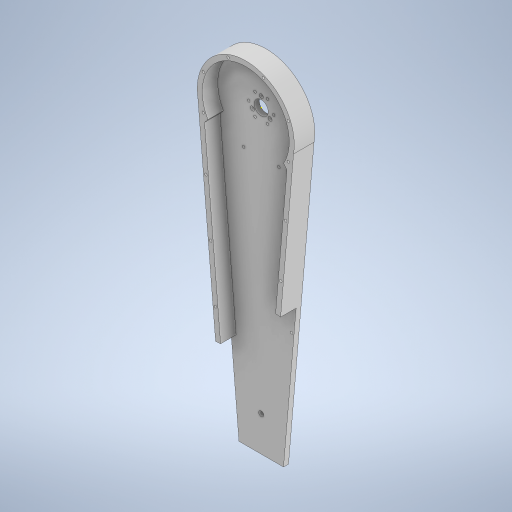
# Autodesk Inventor part: legparts_05(second)
Saved by Autodesk Inventor 2024.3 (Build 283343000, 343)
## iProperties
Created: 2024-10-20
Part Number: legparts_05(second)
Material: 一般
Document SubType Name: Modeling
Designer: 佐藤智貴
Density: 1 g/cm^3
Appearance: 既定
Author: 佐藤智貴
Autodesk Inventor part; units mm, degrees
ref_plane "YZ Plane" through (0, 0, 0) normal (1, 0, 0) x (0, 1, 0)
ref_plane "XZ Plane" through (0, 0, 0) normal (0, 1, 0) x (-1, 0, 0)
ref_plane "XY Plane" through (0, 0, 0) normal (0, 0, 1) x (1, 0, 0)
sketch "スケッチ1" plane through (0, 0, 0) normal (0, 0, 1) x (1, 0, 0)
  circle A0 centre (0, 0) radius 48.5
  circle A1 centre (0, 0) radius 7
  dimension "d0" = 97
  dimension "d1" = 14
  constraints: 2 centre point, 1 coincident
  measures "d0" diameter of A0
  measures "d1" diameter of A1
extrude "押し出し1" add sketch "スケッチ1" along normal blind 20.5
sketch "スケッチ2" plane through (0, 0, 20.5) normal (0, 0, 1) x (1, 0, 0)
  circle A0 centre (0, 0) radius 46
  line L0 (0, 0) -> (0, 59.211)
  line L1 (0, 0) -> (-21.8609, 52.777)
  line L2 (0, 0) -> (27.8226, 47.8581)
  point P0 (-17.6034, 42.4985)
  point P1 (-42.4985, 17.6034)
  point P2 (-42.4985, -17.6034)
  point P3 (-17.6034, -42.4985)
  point P4 (17.6034, -42.4985)
  point P5 (42.4985, -17.6034)
  point P6 (42.4985, 17.6034)
  point P7 (17.6034, 42.4985)
  dimension "d4" = 92
  dimension "d5" = 22.5
  dimension "d8" = 360
  constraints: 6 end point, 1 coincident, 1 point on line, 1 vertical, 12 other
  measures "d5" angle of L1 L0
hole "穴1" at (-17.6034, 42.4985, 20.5) at (-42.4985, 17.6034, 20.5) at (-42.4985, -17.6034, 20.5) at (-17.6034, -42.4985, 20.5) at (17.6034, -42.4985, 20.5) at (42.4985, -17.6034, 20.5) at (42.4985, 17.6034, 20.5) at (17.6034, 42.4985, 20.5) direction (0, 0, -1) diameter 2.459 end through all
sketch "スケッチ3" plane through (0, 0, 20.5) normal (0, 0, 1) x (1, 0, 0)
  circle A0 centre (0, 0) radius 43.5
  dimension "d17" = 87
  constraints: 1 centre point, 1 coincident
  measures "d17" diameter of A0
extrude "押し出し2" cut sketch "スケッチ3" against normal blind 15.5
sketch "スケッチ4" plane through (0, 0, 0) normal (0, 0, -1) x (-1, 0, 0)
  line L0 (0, 0) -> (0, -80.557)
  circle A0 centre (0, 0) radius 48.5 projected
  line L1 (-48.5, 0) -> (-48.5, -300)
  line L2 (48.5, 0) -> (48.5, -300)
  line L3 (-48.5, -300) -> (48.5, -300)
  line L4 (-48.5, 0) -> (-22.2534, -300)
  line L5 (48.5, 0) -> (22.2534, -300)
  point P0 (48.5, 0)
  point P1 (47.7632, -8.4219)
  point P2 (-47.7632, -8.4219)
  dimension "d21" = 48.5
  dimension "d23" = 97
  dimension "d24" = 300
  dimension "d25" = 300
  dimension "d56" = 0
  dimension "d89" = 85
  dimension "d90" = 85
  constraints: 12 end point, 2 point on line, 1 perpendicular, 1 vertical, 2 other
  measures "d21" distance from line of L1 L0.start
  measures "d23" distance between parallel lines of L2 L1
  measures "d24" distance of L2.start L2.end
  measures "d25" distance of L1.start L1.end
  measures "d56" angle of L2 L0
  measures "d89" angle of L3 L5
  measures "d90" angle of L3 L4
extrude "押し出し3" add sketch "スケッチ4" against normal blind 5 contours L5 L3 L4 A0
sketch "スケッチ5" plane through (0, 0, 5) normal (0, 0, 1) x (1, 0, 0)
  line L0 (-48.5, 0) -> (48.5, 0)
  line L1 (-22.2534, -300) -> (22.2534, -300) projected
  circle A0 centre (0, 0) radius 48.5 projected
  circle A1 centre (0, 0) radius 43.5 projected
  line L2 (-47.7632, -8.4219) -> (-22.2534, -300) projected
  line L3 (-48.5, 0) -> (-22.2534, -300)
  line L4 (47.7632, -8.4219) -> (22.2534, -300) projected
  line L5 (-22.2534, -300) -> (22.2534, -300)
  line L6 (22.2534, -300) -> (48.5, 0)
  line L7 (-42.8152, -7.6095) -> (-17.6717, -295)
  line L8 (-17.6717, -295) -> (17.6717, -295)
  line L9 (17.6717, -295) -> (42.7822, -7.9862)
  circle A2 centre (0, 0) radius 48.5
  point P0 (0, -300)
  point P1 (0, -295)
  point P2 (0, -300)
  point P3 (-30.2435, -151.3047)
  point P4 (-41.2491, -25.5101)
  point P5 (41.2491, -25.5101)
  dimension "d33" = 5
  dimension "d91" = 5
  constraints: 14 end point, 3 collinear, 2 midpoint, 1 centre point, 1 coincident, 1 concentric, 2 other
  measures "d33" radial gap between concentric circles of A0 A1
  measures "d91" distance from line of L2 point (-30.243, -151.305)
extrude "押し出し4" add sketch "スケッチ5" along normal blind 15.5 contours L4 L1 L2 A0 L7 L8 L9
sketch "スケッチ6" plane through (0, 0, 20.5) normal (0, 0, 1) x (1, 0, 0)
  line L0 (-22.2534, -300) -> (22.2534, -300) projected
  arc A0 (47.7632, -8.4219) -> (-47.7632, -8.4219) centre (0, 0) ccw projected
  line L1 (-17.6717, -295) -> (-41.2491, -25.5101) projected
  line L2 (41.2491, -25.5101) -> (17.6717, -295) projected
  point P0 (39.8662, -70)
  point P1 (-39.8662, -70)
  point P2 (35.0727, -124.7907)
  point P3 (-35.0727, -124.7907)
  point P4 (30.2791, -179.5814)
  point P5 (-30.2791, -179.5814)
  point P6 (0, -300)
  point P7 (0, 48.5)
  point P8 (48.5, 0)
  dimension "d36" = 348.5
  dimension "d38" = 55
  dimension "d39" = 55
  dimension "d44" = 55
  dimension "d45" = 55
  dimension "d87" = 70
  dimension "d88" = 70
  dimension "d92" = 2.5
  dimension "d93" = 2.5
  dimension "d94" = 2.5
  dimension "d95" = 2.5
  dimension "d96" = 2.5
  dimension "d97" = 2.5
  constraints: 1 midpoint, 1 point on circle
  measures "d36" distance of point (0, -300) point (0, 48.5)
  measures "d38" distance of point (-30.279, -179.581) point (-35.073, -124.791)
  measures "d39" distance of point (-35.073, -124.791) point (-39.866, -70)
  measures "d44" distance of point (30.279, -179.581) point (35.073, -124.791)
  measures "d45" distance of point (39.866, -70) point (35.073, -124.791)
  measures "d87" vertical distance of point (-39.866, -70) point (0, 0)
  measures "d88" vertical distance of point (0, 0) point (39.866, -70)
  measures "d92" distance from line of L1 point (-39.866, -70)
  measures "d93" distance from line of L1 point (-35.073, -124.791)
  measures "d94" distance from line of L1 point (-30.279, -179.581)
  measures "d95" distance from line of L2 point (30.279, -179.581)
  measures "d96" distance from line of L2 point (35.073, -124.791)
  measures "d97" distance from line of L2 point (39.866, -70)
hole "穴2" at (39.8662, -70, 20.5) at (-39.8662, -70, 20.5) at (35.0727, -124.7907, 20.5) at (-35.0727, -124.7907, 20.5) at (30.2791, -179.5814, 20.5) at (-30.2791, -179.5814, 20.5) direction (0, 0, -1) diameter 2.459 end through all
sketch "スケッチ7" plane through (0, 0, 5) normal (0, 0, 1) x (1, 0, 0)
  line L0 (43.5, 0) -> (43.5, -295) projected
  line L1 (43.5, -295) -> (-43.5, -295) projected
  point P0 (0, 0)
  point P1 (0, -265)
  point P2 (48.5, 0)
  dimension "d57" = 43.5
  dimension "d58" = 30
  measures "d57" distance from line of point (0, -265) L0
  measures "d58" distance from line of L1 point (0, -265)
hole "穴3" at (0, -265, 5) direction (0, 0, -1) diameter 5 end through all
sketch "スケッチ12" plane through (0, 0, 20.5) normal (0, 0, 1) x (1, 0, 0)
  circle A0 centre (0, 0) radius 43.5
  circle A1 centre (0, 0) radius 48.5
  line L0 (-41.2491, -25.5101) -> (-17.6717, -295) projected
  line L1 (-41.2491, -25.5101) -> (-37.8431, -21.4511)
  line L2 (17.6717, -295) -> (41.2491, -25.5101) projected
  line L3 (41.2491, -25.5101) -> (37.8431, -21.4511)
  line L4 (-25.9514, -200.3636) -> (-17.1404, -301.073)
  line L5 (-22.2534, -300) -> (-47.7632, -8.4219) projected
  line L6 (-17.1404, -301.073) -> (-22.2534, -300)
  line L7 (-22.2534, -300) -> (-30.1549, -209.6851)
  line L8 (-30.1549, -209.6851) -> (-25.174, -209.2494)
  line L9 (-25.174, -209.2494) -> (-25.9221, -200.6982)
  circle A2 centre (-30.2791, -179.5814) radius 1.2295 projected
  line L10 (22.2534, -300) -> (-22.2534, -300) projected
  line L11 (0, -300) -> (0, -209.4673)
  line L12 (25.9514, -200.3636) -> (17.1404, -301.073)
  line L13 (17.1404, -301.073) -> (22.2534, -300)
  line L14 (22.2534, -300) -> (30.1549, -209.6851)
  line L15 (30.1549, -209.6851) -> (25.174, -209.2494)
  line L16 (25.174, -209.2494) -> (25.9221, -200.6982)
  line L17 (29.8604, -155.6835) -> (34.8413, -156.1193)
  line L18 (47.7632, -8.4219) -> (22.2534, -300) projected
  circle A3 centre (35.0727, -124.7907) radius 1.2295 projected
  line L19 (29.8604, -155.6835) -> (25.174, -209.2494)
  line L20 (34.8413, -156.1193) -> (30.1549, -209.6851)
  line L21 (-17.6717, -295) -> (17.6717, -295)
  line L22 (17.2343, -300) -> (-17.2343, -300)
  point P0 (-27.6644, -209.4673)
  point P1 (27.6644, -209.4673)
  point P2 (32.3508, -155.9014)
  dimension "d98" = 87
  dimension "d99" = 97
  dimension "d100" = 135
  dimension "d101" = 135
  dimension "d102" = 30
  dimension "d106" = 30
  constraints: 36 end point, 12 point on line, 6 symmetric about line, 3 midpoint, 2 centre point, 2 coincident, 2 point on circle, 1 collinear, 1 horizontal, 1 parallel, 1 perpendicular, 1 vertical
  measures "d98" diameter of A0
  measures "d99" diameter of A1
  measures "d100" angle of L0 L1
  measures "d101" angle of L2 L3
  measures "d102" distance of point (-27.664, -209.467) A2.centre
  measures "d106" distance edge to line of A3 L17
extrude "押し出し9" cut sketch "スケッチ12" against normal blind 15.5 contours A0 L3 A1 L1 | L17 L18 L15 L2 | L8 L0 L4 L10 L5 | L10 L4 L6 | L14 L10 L12 L2 L15 | L4 L21 L11 L10 | L11 L21 L12 L10 picked at (4.5296, -44.776)
sketch "スケッチ13" plane through (0, 0, 5) normal (0, 0, 1) x (1, 0, 0)
  circle A0 centre (0, 0) radius 43.5
  circle A1 centre (0, 0) radius 12.5
  line L0 (0, 0) -> (-7.2545, 12.5652)
  line L1 (0, 0) -> (0, 17.1386)
  point P0 (-6.25, 10.8253)
  point P1 (-12.5, 0)
  point P2 (-6.25, -10.8253)
  point P3 (6.25, -10.8253)
  point P4 (12.5, 0)
  point P5 (6.25, 10.8253)
  dimension "d110" = 25
  dimension "d107" = 87
  dimension "d111" = 30
  dimension "d112" = 360
  constraints: 4 end point, 2 coincident, 1 centre point, 1 point on line, 1 vertical, 10 other
  measures "d107" diameter of A0
  measures "d111" angle of L1 L0
hole "穴4" at (-6.25, 10.8253, 5) at (6.25, 10.8253, 5) at (12.5, 0, 5) at (6.25, -10.8253, 5) at (-6.25, -10.8253, 5) at (-12.5, 0, 5) direction (0, 0, -1) diameter 2.459 depth 8 tip angle 118
sketch "スケッチ14" plane through (0, 0, 5) normal (0, 0, 1) x (1, 0, 0)
  circle A0 centre (0, 0) radius 10.2
  point P0 (0.0737, 10.1997)
  point P1 (0.0737, 10.1997)
  point P2 (-8.8701, -5.036)
  point P3 (8.7964, -5.1637)
  dimension "d122" = 20.4
  dimension "d123" = 360
  constraints: 3 coincident, 7 other
hole "穴5" at (0.0737, 10.1997, 5) at (8.7964, -5.1637, 5) at (-8.8701, -5.036, 5) direction (0, 0, -1) diameter 4 depth 8 tip angle 118
sketch "スケッチ15" plane through (0, 0, 5) normal (0, 0, 1) x (1, 0, 0)
  point P0 (0, 0)
equation "\"d25\" = d24"
equation "\"d90\" = d89"
equation "\"d44\" = d43"
equation "\"d45\" = d44"
equation "\"d88\" = d87"
equation "\"d93\" = d92"
equation "\"d94\" = d93"
equation "\"d95\" = d94"
equation "\"d96\" = d93"
equation "\"d97\" = d92"
equation "\"d57\" = 0.5 * d86"
equation "\"d43\" = d37"
equation "\"d37\" = 55"
equation "\"d86\" = 87"
